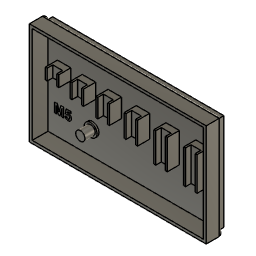
M5 Reference Caliper From 6 v2 (Autodesk Fusion 360 design; units mm, degrees)
Autodesk Fusion 360 part; units mm, degrees
note: some values were not read from the file. Chosen so that the rebuilt part matches the saved one: which bodies a step acts on; which pieces of a blend or face edit are solid.
sketch "Schizzo1" plane through (0, 0, 0) normal (0, 1, 0) x (1, 0, 0)
  line L0 (-43.0702, -47.1256) -> (51.9298, -47.1256)
  line L1 (51.9298, -47.1256) -> (51.9298, 7.8744)
  line L2 (51.9298, 7.8744) -> (-43.0702, 7.8744)
  line L3 (-43.0702, 7.8744) -> (-43.0702, -47.1256)
  line L4 (-34.9398, -37.8859) -> (-30.6504, -37.8859) construction
  line L5 (-30.6504, -37.8859) -> (-30.6504, -43.5032) construction
  line L6 (-30.6504, -43.5032) -> (-34.9398, -43.5032) construction
  line L7 (-34.9398, -43.5032) -> (-34.9398, -37.8859) construction
  line L8 (-20.4362, -37.8859) -> (-16.447, -37.8859) construction
  line L9 (-16.447, -37.8859) -> (-16.447, -43.5032) construction
  line L10 (-16.447, -43.5032) -> (-20.4362, -43.5032) construction
  line L11 (-20.4362, -43.5032) -> (-20.4362, -37.8859) construction
  line L12 (-8.7087, -37.8859) -> (-3.8667, -37.8859) construction
  line L13 (-3.8667, -37.8859) -> (-3.8667, -43.5032) construction
  line L14 (-3.8667, -43.5032) -> (-8.7087, -43.5032) construction
  line L15 (-8.7087, -43.5032) -> (-8.7087, -37.8859) construction
  line L16 (7.3795, -37.8859) -> (14.0192, -37.8859) construction
  line L17 (14.0192, -37.8859) -> (14.0192, -43.5032) construction
  line L18 (14.0192, -43.5032) -> (7.3795, -43.5032) construction
  line L19 (7.3795, -43.5032) -> (7.3795, -37.8859) construction
  line L20 (21.7115, -37.8859) -> (29.1532, -37.8859) construction
  line L21 (29.1532, -37.8859) -> (29.1532, -43.5032) construction
  line L22 (29.1532, -43.5032) -> (21.7115, -43.5032) construction
  line L23 (21.7115, -43.5032) -> (21.7115, -37.8859) construction
  line L24 (-36.48, -29.271) -> (-29.28, -29.271)
  line L25 (-29.28, -29.271) -> (-29.28, -23.271)
  line L26 (-29.28, -23.271) -> (-36.48, -23.271)
  line L27 (-36.48, -23.271) -> (-36.48, -29.271)
  line L28 (-32.88, -29.271) -> (-32.88, -23.271) construction
  line L29 (-30.28, -23.271) -> (-35.48, -23.271)
  line L30 (-35.48, -23.271) -> (-35.48, -29.271)
  line L31 (-35.48, -29.271) -> (-30.28, -29.271)
  line L32 (-30.28, -29.271) -> (-30.28, -23.271)
  line L33 (-30.28, -23.271) -> (-35.48, -29.271) construction
  line L34 (-35.48, -23.271) -> (-30.28, -29.271) construction
  line L35 (-15.9419, -21.271) -> (-23.1419, -21.271)
  line L36 (-22.1419, -21.271) -> (-16.9419, -29.271) construction
  line L37 (-16.9419, -21.271) -> (-22.1419, -21.271)
  line L38 (-16.9419, -29.271) -> (-16.9419, -21.271)
  line L39 (-22.1419, -21.271) -> (-22.1419, -29.271)
  line L40 (-16.9419, -21.271) -> (-22.1419, -29.271) construction
  line L41 (-19.5419, -29.271) -> (-19.5419, -21.271) construction
  line L42 (-23.1419, -29.271) -> (-15.9419, -29.271)
  line L43 (-23.1419, -21.271) -> (-23.1419, -29.271)
  line L44 (-15.9419, -29.271) -> (-15.9419, -21.271)
  line L45 (-22.1419, -29.271) -> (-16.9419, -29.271)
  line L46 (-3.0584, -29.271) -> (-3.0584, -19.271)
  line L47 (-9.2584, -19.271) -> (-9.2584, -29.271)
  line L48 (-2.0584, -29.271) -> (-2.0584, -19.271)
  line L49 (-9.2584, -29.271) -> (-2.0584, -29.271)
  line L50 (-3.0584, -19.271) -> (-8.2584, -29.271) construction
  line L51 (-3.0584, -19.271) -> (-8.2584, -19.271)
  line L52 (-8.2584, -19.271) -> (-8.2584, -29.271)
  line L53 (-8.2584, -19.271) -> (-3.0584, -29.271) construction
  line L54 (-2.0584, -19.271) -> (-9.2584, -19.271)
  line L55 (-5.6584, -29.271) -> (-5.6584, -19.271) construction
  line L56 (-8.2584, -29.271) -> (-3.0584, -29.271)
  line L57 (6.8674, -29.271) -> (12.0674, -29.271)
  line L58 (6.8674, -17.271) -> (6.8674, -29.271)
  line L59 (5.8674, -29.271) -> (13.0674, -29.271)
  line L60 (12.0674, -29.271) -> (12.0674, -17.271)
  line L61 (12.0674, -17.271) -> (6.8674, -29.271) construction
  line L62 (13.0674, -17.271) -> (5.8674, -17.271)
  line L63 (9.4674, -29.271) -> (9.4674, -17.271) construction
  line L64 (5.8674, -17.271) -> (5.8674, -29.271)
  line L65 (12.0674, -17.271) -> (6.8674, -17.271)
  line L66 (6.8674, -17.271) -> (12.0674, -29.271) construction
  line L67 (13.0674, -29.271) -> (13.0674, -17.271)
  line L68 (-43.0702, -29.271) -> (51.9298, -29.271) construction
  line L69 (21.8159, -29.271) -> (29.0159, -29.271)
  line L70 (28.0159, -13.271) -> (22.8159, -29.271) construction
  line L71 (29.0159, -29.271) -> (29.0159, -13.271)
  line L72 (21.8159, -13.271) -> (21.8159, -29.271)
  line L73 (28.0159, -29.271) -> (28.0159, -13.271)
  line L74 (28.0159, -13.271) -> (22.8159, -13.271)
  line L75 (25.4159, -29.271) -> (25.4159, -13.271) construction
  line L76 (22.8159, -13.271) -> (22.8159, -29.271)
  line L77 (22.8159, -29.271) -> (28.0159, -29.271)
  line L78 (22.8159, -13.271) -> (28.0159, -29.271) construction
  line L79 (29.0159, -13.271) -> (21.8159, -13.271)
  line L80 (-43.0702, -43.5032) -> (51.9298, -43.5032) construction
  line L81 (50.4298, -45.6256) -> (50.4298, 6.3744)
  line L82 (50.4298, 6.3744) -> (-41.5702, 6.3744)
  line L83 (-41.5702, 6.3744) -> (-41.5702, -45.6256)
  line L84 (-41.5702, -45.6256) -> (50.4298, -45.6256)
  line L85 (-38, -4) -> (-25, -4) construction
  line L86 (-25, -4) -> (-25, -9) construction
  line L87 (-25, -9) -> (-38, -9) construction
  line L88 (-38, -9) -> (-38, -4) construction
  line L89 (-43.0702, -37.8859) -> (50.4298, -37.8859) construction
  circle A0 centre (-17.6815, -6.6421) radius 2.5
  circle A1 centre (-17.6815, -6.6421) radius 3.5
  line L90 (37.7115, -37.8859) -> (45.1532, -37.8859) construction
  line L91 (45.1532, -37.8859) -> (45.1532, -43.5032) construction
  line L92 (45.1532, -43.5032) -> (37.7115, -43.5032) construction
  line L93 (37.7115, -43.5032) -> (37.7115, -37.8859) construction
  line L94 (41.4209, -29.271) -> (41.4209, -11.271) construction
  line L95 (44.0209, -11.271) -> (38.8209, -11.271)
  line L96 (38.8209, -11.271) -> (38.8209, -29.271)
  line L97 (38.8209, -29.271) -> (44.0209, -29.271)
  line L98 (44.0209, -29.271) -> (44.0209, -11.271)
  line L99 (44.0209, -11.271) -> (38.8209, -29.271) construction
  line L100 (38.8209, -11.271) -> (44.0209, -29.271) construction
  line L101 (37.8209, -29.271) -> (45.0209, -29.271)
  line L102 (45.0209, -29.271) -> (45.0209, -11.271)
  line L103 (45.0209, -11.271) -> (37.8209, -11.271)
  line L104 (37.8209, -11.271) -> (37.8209, -29.271)
  line L105 (41.4209, -29.271) -> (41.4209, -11.271) construction
  point P0 (-32.88, -26.271)
  point P1 (-19.5419, -25.271)
  point P2 (-5.6584, -24.271)
  point P3 (9.4674, -23.271)
  point P4 (25.4159, -21.271)
  point P5 (41.4209, -20.271)
  dimension "d1" = 55
  dimension "d2" = 5
  dimension "d3" = 5
  dimension "d4" = 5
  dimension "d5" = 5
  dimension "d6" = 5
  dimension "d7" = 7.2
  dimension "d8" = 6
  dimension "d9" = 5.2
  dimension "d21" = 7.2
  dimension "d22" = 8
  dimension "d23" = 5.2
  dimension "d24" = 7.2
  dimension "d25" = 10
  dimension "d26" = 5.2
  dimension "d27" = 7.2
  dimension "d28" = 12
  dimension "d29" = 5.2
  dimension "d30" = 7.2
  dimension "d31" = 16
  dimension "d32" = 5.2
  dimension "d33" = 95
  dimension "d34" = -1.5
  dimension "d37" = 5
  dimension "d40" = 5
  dimension "d41" = 7
  dimension "d50" = 5
  dimension "d53" = 5.2
  dimension "d54" = 18
  dimension "d55" = 7.2
  text T0 "6" font "Arial" height 5 bold align left middle in box 4.2894 x 5.6173 at (-34.9398, -37.8859) x (1, 0) y (0, -1) spacing 1
  text T1 "8" font "Arial" height 5 bold align left top in box 3.9891 x 5.6173 at (-20.4362, -37.8859) x (1, 0) y (0, -1) spacing 1
  text T2 "10\n" font "Arial" height 5 bold align left top in box 4.842 x 5.6173 at (-8.7087, -37.8859) x (1, 0) y (0, -1) spacing 1
  text T3 "12" font "Arial" height 5 bold align left top in box 6.6397 x 5.6173 at (7.3795, -37.8859) x (1, 0) y (0, -1) spacing 1
  text T4 "16" font "Arial" height 5 bold align left top in box 7.4417 x 5.6173 at (21.7115, -37.8859) x (1, 0) y (0, -1) spacing 1
  text T5 "M5" font "Arial" height 5 bold align left top in box 13 x 5 at (-38, -4) x (1, 0) y (0, -1) spacing 1
  text T6 "18" font "Arial" height 5 bold align left top in box 7.4417 x 5.6173 at (37.7115, -37.8859) x (1, 0) y (0, -1) spacing 1
  constraint horizontal L0
  constraint vertical L1
  constraint horizontal L2
  constraint vertical L3
  constraint horizontal L24
  constraint vertical L25
  constraint horizontal L26
  constraint vertical L27
  constraint midpoint L24 L28.start
  constraint midpoint L26 L28.end
  constraint horizontal L29
  constraint perpendicular L29 L30
  constraint parallel L29 L31
  constraint parallel L30 L32
  constraint coincident L33 P0
  constraint coincident L34 P0
  constraint coincident L26 L29.start
  constraint midpoint L28 P0
  constraint horizontal L42
  constraint vertical L44
  constraint horizontal L35
  constraint vertical L43
  constraint midpoint L41.start L42
  constraint midpoint L41.end L35
  constraint horizontal L37
  constraint perpendicular L37 L39
  constraint parallel L37 L45
  constraint parallel L38 L39
  constraint coincident P1 L40
  constraint coincident P1 L36
  constraint coincident L37.start L35
  constraint midpoint P1 L41
  constraint horizontal L49
  constraint vertical L48
  constraint horizontal L54
  constraint vertical L47
  constraint midpoint L55.start L49
  constraint midpoint L55.end L54
  constraint horizontal L51
  constraint perpendicular L51 L52
  constraint parallel L51 L56
  constraint parallel L46 L52
  constraint coincident P2 L50
  constraint coincident P2 L53
  constraint coincident L46.end L54
  constraint midpoint P2 L55
  constraint horizontal L59
  constraint vertical L67
  constraint horizontal L62
  constraint vertical L64
  constraint midpoint L63.start L59
  constraint midpoint L63.end L62
  constraint horizontal L65
  constraint perpendicular L58 L65
  constraint parallel L57 L65
  constraint parallel L58 L60
  constraint coincident P3 L61
  constraint coincident P3 L66
  constraint coincident L60.end L62
  constraint midpoint P3 L63
  constraint coincident L3 L68.start
  constraint coincident L1 L68.end
  constraint perpendicular L1 L68
  constraint collinear L31 L68
  constraint collinear L49 L68
  constraint collinear L59 L68
  constraint horizontal L69
  constraint vertical L71
  constraint horizontal L79
  constraint vertical L72
  constraint midpoint L75.start L69
  constraint midpoint L75.end L79
  constraint horizontal L74
  constraint perpendicular L74 L76
  constraint parallel L74 L77
  constraint parallel L73 L76
  constraint coincident P4 L70
  constraint coincident P4 L78
  constraint coincident L70.start L79
  constraint midpoint P4 L75
  constraint coincident L3 L80.start
  constraint coincident L1 L80.end
  constraint perpendicular L1 L80
  constraint collinear L42 L68
  constraint collinear L68 L69
  constraint collinear L6 L80
  constraint collinear L10 L80
  constraint collinear L14 L80
  constraint collinear L18 L80
  constraint collinear L22 L80
  constraint coincident L3 L89.start
  constraint coincident L81 L89.end
  constraint perpendicular L81 L89
  constraint collinear L4 L89
  constraint collinear L8 L89
  constraint collinear L12 L89
  constraint collinear L16 L89
  constraint collinear L20 L89
  constraint concentric A0 A1
  constraint coincident L68 L94.start
  constraint perpendicular L68 L94
  constraint horizontal L95
  constraint perpendicular L95 L96
  constraint parallel L95 L97
  constraint parallel L96 L98
  constraint coincident L99 P5
  constraint coincident L100 P5
  constraint midpoint L94 P5
  constraint horizontal L101
  constraint vertical L102
  constraint horizontal L103
  constraint vertical L104
  constraint collinear L68 L101
  constraint collinear L68 L97
  constraint collinear L95 L103
  constraint midpoint L101 L94.start
  constraint midpoint L103 L94.end
  constraint collinear L94 L105
  measures "d1" distance of L0 L2
  measures "d7" distance of L24.start L24.end
  measures "d8" distance of L24.start L26.end
  measures "d9" distance of L30 L32
  measures "d21" distance of L42.start L42.end
  measures "d22" distance of L42.start L35.end
  measures "d23" distance of L38 L39
  measures "d24" distance of L47.end L48.start
  measures "d25" distance of L47.start L47.end
  measures "d26" distance of L46 L52
  measures "d27" distance of L59.end L59.start
  measures "d28" distance of L62.end L59.start
  measures "d29" distance of L58 L60
  measures "d30" distance of L69.start L69.end
  measures "d31" distance of L69.start L72.start
  measures "d32" distance of L73 L76
  measures "d33" distance of L1 L3
  measures "d40" diameter of A0
  measures "d41" diameter of A1
  measures "d53" distance of L96.end L97.end
  measures "d54" distance of L95.end L96.end
  measures "d55" distance of L102 L104
extrude "Estrusione1" add sketch "Schizzo1" along normal blind 0.4 text T0 T1 T2 T3 T4 T5 T6 makes body 1 at (-34.2253, 0, 40.6556) makes body 2 at (26.055, 0, 40.9643) makes body 3 at (-2.1808, 0, 40.6141) makes body 4 at (-18.3806, 0, 41.1837) makes body 5 at (12.491, 0, 38.8) makes body 6 at (23.5885, 0, 41.3807) makes body 7 at (-31.7301, 0, 7.4823) makes body 8 at (-37.6874, 0, 6.9786) makes body 9 at (-6.8317, 0, 41.3807) makes body 10 at (9.2565, 0, 41.3807) makes body 11 at (43.3824, 0, 41.1837) makes body 12 at (39.5885, 0, 41.3807)
extrude "Estrusione2" add sketch "Schizzo1" along normal blind 0.5 separate body contours L0 L1 L2 L3 | L24 L26 L27 L30 | L24 L26 L29 L30 L31 L32 | L24 L25 L26 L32 | L35 L38 L42 L44 | L35 L37 L38 L39 L42 L45 | L35 L39 L42 L43 | L46 L49 L51 L52 L54 L56 | L46 L48 L49 L54 | L47 L49 L52 L54 | L57 L58 L59 L60 L62 L65 | L58 L59 L62 L64 | L59 L60 L62 L67 | L69 L72 L76 L79 | L69 L73 L74 L76 L77 L79 | L69 L71 L73 L79 | L81 L82 L83 L84 | A0 | A1 | L95 L96 L97 L98 L101 L103 | L98 L101 L102 L103 | L96 L101 L103 L104 makes body 13
extrude "Estrusione7" cut sketch "Schizzo1" 2 faces at (39.5885, 0, 41.3807) (43.3824, 0, 41.1837) along normal blind 0.4 text T0 T1 T2 T3 T5 T4 on bodies 11 12 bodies 13
extrude "Estrusione6" add sketch "Schizzo1" against normal blind 8.5 contours L0 L1 L2 L3 bodies 13
extrude "Estrusione4" add sketch "Schizzo1" against normal blind 6.5 contours L24 L26 L27 L30 | L24 L26 L29 L30 L31 L32 | L24 L25 L26 L32 | L35 L38 L42 L44 | L35 L37 L38 L39 L42 L45 | L35 L39 L42 L43 | L46 L49 L51 L52 L54 L56 | L46 L48 L49 L54 | L47 L49 L52 L54 | L57 L58 L59 L60 L62 L65 | L58 L59 L62 L64 | L59 L60 L62 L67 | L69 L72 L76 L79 | L69 L73 L74 L76 L77 L79 | L69 L71 L73 L79 | A0 | L95 L96 L97 L98 L101 L103 | L98 L101 L102 L103 | L96 L101 L103 L104 bodies 13
extrude "Estrusione8" add sketch "Schizzo1" against normal blind 1 contours A1 bodies 13
extrude "Estrusione5" cut sketch "Schizzo1" along normal blind 3 from surface at -6.5 contours L24 L26 L29 L30 L31 L32 | L35 L37 L38 L39 L42 L45 | L46 L49 L51 L52 L54 L56 | L57 L58 L59 L60 L62 L65 | L69 L73 L74 L76 L77 L79 | L95 L96 L97 L98 L101 L103 bodies 13
sketch "Schizzo2" plane through (0, 0.5, 0) normal (0, 1, 0) x (-1, 0, 0)
  line L0 (43.0702, -7.8744) -> (43.0702, 47.1256)
  line L1 (43.0702, 47.1256) -> (-51.9298, 47.1256)
  line L2 (-51.9298, 47.1256) -> (-51.9298, -7.8744)
  line L3 (-51.9298, -7.8744) -> (43.0702, -7.8744)
  line L4 (-51.9298, 47.1256) -> (43.0702, 47.1256) construction
  line L5 (43.0702, 47.1256) -> (43.0702, -7.8744) construction
  line L6 (43.0702, -7.8744) -> (-51.9298, -7.8744) construction
  line L7 (-51.9298, -7.8744) -> (-51.9298, 47.1256) construction
  line L8 (-51.9298, 19.6256) -> (-50, 19.6256) construction
  line L9 (-50, 19.6256) -> (43.0702, 19.6256) construction
  line L10 (-4.4298, 47.1256) -> (-4.4298, -7.8744) construction
  line L11 (41.5702, -6.3744) -> (-50.4298, -6.3744)
  line L12 (-50.4298, -6.3744) -> (-50.4298, 45.6256)
  line L13 (-50.4298, 45.6256) -> (41.5702, 45.6256)
  line L14 (41.5702, 45.6256) -> (41.5702, -6.3744)
  line L15 (41.5702, -6.3744) -> (-50.4298, 45.6256) construction
  line L16 (-50.4298, -6.3744) -> (41.5702, 45.6256) construction
  point P0 (-4.4298, 19.6256)
  dimension "d44" = 1.5
  dimension "d45" = 1.5
  constraint horizontal L4
  constraint vertical L5
  constraint horizontal L6
  constraint vertical L7
  constraint coincident L0.end L1.start
  constraint coincident L2.end L3.start
  constraint midpoint L7 L8.start
  constraint perpendicular L7 L8
  constraint midpoint L5 L9.end
  constraint perpendicular L5 L9
  constraint midpoint L4 L10.start
  constraint midpoint L6 L10.end
  constraint horizontal L11
  constraint perpendicular L11 L12
  constraint parallel L11 L13
  constraint parallel L12 L14
  constraint coincident L15 P0
  constraint coincident L16 P0
  constraint midpoint L10 P0
  measures "d44" distance of L7 L12
  measures "d45" distance of L4 L13
extrude "Estrusione9" add sketch "Schizzo2" along normal blind 2 contours L11 L12 L13 L14 bodies 13
fillet "Raccordo1" radius 2 4 edges at (51.9298, 0.5, 19.6256) (4.4298, 0.5, -7.8744) (-43.0702, 0.5, 19.6256) (4.4298, 0.5, 47.1256) on bodies 13
equation "d7 = d9 + 2 mm"
equation "d21 = d7"
equation "d23 = d9"
equation "d24 = d7"
equation "d26 = d9"
equation "d27 = d7"
equation "d29 = d9"
equation "d30 = d7"
equation "d32 = d9"
equation "d41 = d40 + 2 mm"
equation "d45 = d44"
equation "d53 = d9"
equation "d55 = d7"
